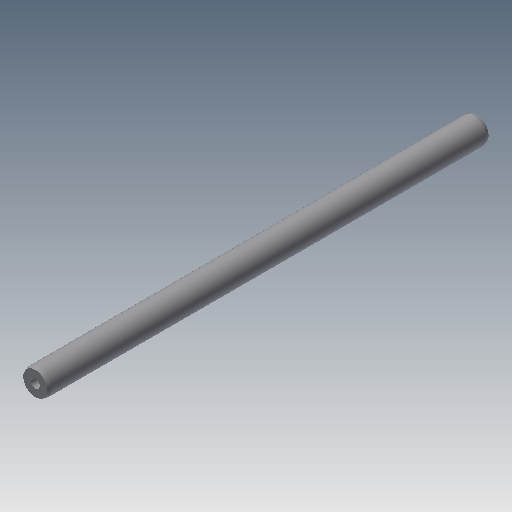
# Autodesk Inventor part: ER4_CageRod
Saved by Autodesk Inventor 2019 (Build 230136000, 136)
## iProperties
Created: 2014-02-10
Part Number: ER4_CageRod
Material: Generic
Document SubType Name: Modeling
Designer: voigt
Density: 1 g/cm^3
Appearance: Default
Author: voigt
Autodesk Inventor part; units mm, degrees
ref_plane "YZ Plane" through (0, 0, 0) normal (1, 0, 0) x (0, 1, 0)
ref_plane "XZ Plane" through (0, 0, 0) normal (0, 1, 0) x (-1, 0, 0)
ref_plane "XY Plane" through (0, 0, 0) normal (0, 0, 1) x (1, 0, 0)
sketch "Sketch1" plane through (0, 0, 0) normal (0, 0, 1) x (1, 0, 0)
  circle A0 centre (0, 0) radius 3
  dimension "d0" = 6
  constraints: 1 centre point, 1 coincident
  measures "d0" diameter of A0
extrude "Extrusion1" add sketch "Sketch1" along normal blind 101.6
chamfer "Chamfer1" distance 0.254 distance2 0.762 1 edges at (-3, 0, 0) measured on face at (-0.5351, 1.0949, 0)
chamfer "Chamfer2" distance 0.254 distance2 0.762 1 edges at (-3, 0, 101.6) measured on face at (-0.5351, 1.0949, 101.6)
sketch "Sketch2" plane through (0, 0, 0) normal (0, 0, -1) x (-1, 0, 0)
  circle A0 centre (0, 0) radius 2.746 projected
  constraints: 1 coincident
sketch "Sketch3" plane through (0, 0, 101.6) normal (0, 0, 1) x (1, 0, 0)
  circle A0 centre (0, 0) radius 2.746 projected
  constraints: 1 coincident
hole "Hole1" at (0, 0, 0) direction (0, 0, 1) diameter 2.156 depth 5 tip angle 118
hole "Hole2" at (0, 0, 101.6) direction (0, 0, -1) diameter 2.156 depth 5 tip angle 118
body "Solid1"
